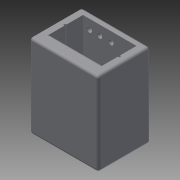
# Autodesk Inventor part: Part1
Saved by Autodesk Inventor 2014 SP1 (Build 180222100, 222)
## iProperties
Created: 2013-12-01
Part Number: Part1
Material: Generic
Document SubType Name: Modeling
Designer: Tim
Density: 1 g/cm^3
Appearance: Default
Author: Tim
Autodesk Inventor part; units mm, degrees
ref_plane "YZ Plane" through (0, 0, 0) normal (1, 0, 0) x (0, 1, 0)
ref_plane "XZ Plane" through (0, 0, 0) normal (0, 1, 0) x (-1, 0, 0)
ref_plane "XY Plane" through (0, 0, 0) normal (0, 0, 1) x (1, 0, 0)
sketch "Sketch1" plane through (0, 0, 0) normal (0, 1, 0) x (-1, 0, 0)
  line L0 (27.4909, -23.2831) -> (-26.5091, -23.2831)
  line L1 (-26.5091, -23.2831) -> (-26.5091, 42.2169)
  line L2 (-26.5091, 42.2169) -> (27.4909, 42.2169)
  line L3 (27.4909, 42.2169) -> (27.4909, -23.2831)
  point P0 (0, 0)
  dimension "d0" = 54
  dimension "d1" = 65.5
  constraints: 8 end point, 2 parallel, 1 horizontal, 1 perpendicular
  measures "d0" distance between parallel lines of L3 L1
  measures "d1" distance between parallel lines of L0 L2
extrude "Extrusion1" add sketch "Sketch1" along normal blind 41
sketch "Sketch2" plane through (-27.4909, 0, 42.2169) normal (0, 0, 1) x (1, 0, 0)
  line L0 (54, 0) -> (0, 0) projected
  line L1 (54, 0) -> (54, 41) projected
  line L2 (0, 41) -> (54, 41) projected
  line L3 (0, 0) -> (0, 41) projected
  line L4 (6, 36) -> (48, 36)
  line L5 (48, 36) -> (48, 5)
  line L6 (48, 5) -> (6, 5)
  line L7 (6, 5) -> (6, 36)
  line L8 (5, 23) -> (49, 23)
  line L9 (49, 23) -> (49, 21.5)
  line L10 (49, 21.5) -> (5, 21.5)
  line L11 (5, 21.5) -> (5, 23)
  point P0 (27.4909, 0)
  dimension "d4" = 42
  dimension "d5" = 31
  dimension "d6" = 5
  dimension "d7" = 6
  dimension "d8" = 6
  dimension "d9" = 1
  dimension "d10" = 1
  dimension "d11" = 13
  dimension "d12" = 1.5
  dimension "d13" = 5
  constraints: 16 end point, 4 parallel, 2 horizontal, 2 perpendicular
  measures "d4" distance between parallel lines of L5 L7
  measures "d5" distance between parallel lines of L6 L4
  measures "d6" distance between parallel lines of L4 L2
  measures "d7" distance between parallel lines of L1 L5
  measures "d8" distance between parallel lines of L3 L7
  measures "d9" distance between parallel lines of L7 L11
  measures "d10" distance between parallel lines of L9 L5
  measures "d11" distance between parallel lines of L4 L8
  measures "d12" distance between parallel lines of L8 L10
  measures "d13" distance between parallel lines of L0 L6
extrude "Extrusion2" cut sketch "Sketch2" against normal blind 60.5 contours L4 L5 L8 L7 | L8 L5 L10 L7 | L7 L10 L11 L8 | L8 L9 L10 L5 | L10 L5 L6 L7
sketch "Sketch3" plane through (0, 41, 0) normal (0, 1, 0) x (1, 0, 0)
  line L0 (26.5091, 23.2831) -> (-27.4909, 23.2831) projected
  line L1 (26.5091, -42.2169) -> (26.5091, 23.2831) projected
  line L2 (-7.9909, -6.7169) -> (19.5091, -6.7169)
  line L3 (19.5091, -6.7169) -> (19.5091, 16.2831)
  line L4 (19.5091, 16.2831) -> (-7.9909, 16.2831)
  line L5 (-7.9909, 16.2831) -> (-7.9909, -6.7169)
  point P0 (0, 0)
  dimension "d16" = 34.5
  dimension "d17" = 30
  dimension "d18" = 7
  dimension "d19" = 7
  constraints: 8 end point, 2 parallel, 1 horizontal, 1 perpendicular
  measures "d16" distance between parallel lines of L1 L5
  measures "d17" distance between parallel lines of L0 L2
  measures "d18" distance between parallel lines of L0 L4
  measures "d19" distance between parallel lines of L1 L3
extrude "Extrusion3" cut sketch "Sketch3" against normal blind 5
sketch "Sketch4" plane through (-21.4909, 5, 42.2169) normal (0, 1, 0) x (1, 0, 0)
  line L0 (0, 0) -> (0, 60.5) projected
  line L1 (0, 3) -> (42, 3)
  line L2 (42, 3) -> (42, 0)
  line L3 (42, 0) -> (0, 0)
  line L4 (0, 0) -> (0, 3)
  point P0 (21.4909, 42.2169)
  dimension "d22" = 3
  constraints: 8 end point, 2 parallel, 1 horizontal, 1 perpendicular, 1 point on line
  measures "d22" distance between parallel lines of L3 L1
extrude "Extrusion4" add sketch "Sketch4" along normal blind 5 separate body
sketch "Sketch5" plane through (0, 41, 0) normal (0, 1, 0) x (1, 0, 0)
  line L0 (26.5091, 23.2831) -> (-27.4909, 23.2831) projected
  line L1 (-27.4909, 23.2831) -> (-27.4909, -42.2169) projected
  circle A0 centre (-16.4909, -34.7169) radius 2
  circle A1 centre (-8.4909, -34.7169) radius 2
  circle A2 centre (0.5091, -34.7169) radius 2
  point P0 (0, 0)
  dimension "d25" = 11
  dimension "d26" = 19
  dimension "d27" = 28
  dimension "d30" = 58
  dimension "d31" = 58
  dimension "d32" = 58
  dimension "d33" = 4
  dimension "d34" = 4
  dimension "d35" = 4
  constraints: 3 centre point
  measures "d25" distance from line of L1 A0.centre
  measures "d26" distance from line of A1.centre L1
  measures "d27" distance from line of A2.centre L1
  measures "d30" distance from line of L0 A0.centre
  measures "d31" distance from line of L0 A1.centre
  measures "d32" distance from line of L0 A2.centre
  measures "d33" diameter of A1
  measures "d34" diameter of A2
  measures "d35" diameter of A0
extrude "Extrusion5" cut sketch "Sketch5" against normal blind 5 bodies 1
fillet "Fillet3" radius 2 1 edges at (26.5091, 20.5, -23.2831)
fillet "Fillet4" radius 2 1 edges at (-27.4909, 20.5, -23.2831)
fillet "Fillet5" radius 2 5 edges at (-0.4909, 41, -23.2831) (-26.9051, 41, -22.6973) (-27.4909, 41, 10.4669) (25.9233, 41, -22.6973) (26.5091, 41, 10.4669)
fillet "Fillet6" radius 2 5 edges at (-0.4909, 0, -23.2831) (25.9233, 0, -22.6973) (26.5091, 0, 10.4669) (-26.9051, 0, -22.6973) (-27.4909, 0, 10.4669)
fillet "Fillet7" radius 2 8 edges at (-27.4909, 20.5, 42.2169) (-26.9051, 40.4142, 42.2169) (-0.4909, 41, 42.2169) (25.9233, 40.4142, 42.2169) (26.5091, 20.5, 42.2169) (25.9233, 0.5858, 42.2169) (-0.4909, 0, 42.2169) (-26.9051, 0.5858, 42.2169)
fillet "Fillet9" radius 1 3 edges at (-10.4909, 41, 34.7169) (-1.4909, 41, 34.7169) (-18.4909, 41, 34.7169)
fillet "Fillet11" radius 2 1 edges at (-0.4909, 10, 42.2169)
sketch "Sketch6" plane through (24.5091, 39, -23.2831) normal (0, 0, -1) x (-1, 0, 0)
  line L0 (50, 0) -> (50, -37) projected
  line L1 (0, 0) -> (50, 0) projected
  line L2 (0, -37) -> (0, 0) projected
  line L3 (3, -10) -> (47, -10) construction
  line L4 (47, -10) -> (47, -27) construction
  line L5 (47, -27) -> (3, -27) construction
  line L6 (3, -27) -> (3, -10) construction
  line L7 (5.0416, -16.1395) -> (5.0416, -10.7613)
  line L8 (5.0416, -10.7613) -> (2.9951, -10.7613)
  line L9 (2.9951, -10.7613) -> (2.9951, -10.0395)
  line L10 (2.9951, -10.0395) -> (7.8988, -10.0395)
  line L11 (7.8988, -10.0395) -> (7.8988, -10.7613)
  line L12 (7.8988, -10.7613) -> (5.8523, -10.7613)
  line L13 (5.8523, -10.7613) -> (5.8523, -16.1395)
  line L14 (5.8523, -16.1395) -> (5.0416, -16.1395)
  line L15 (9.2434, -16.1395) -> (8.4722, -16.1395)
  line L16 (8.4722, -16.1395) -> (8.4722, -11.5621)
  line L17 (8.4722, -11.5621) -> (9.2434, -11.5621)
  line L18 (9.2434, -11.5621) -> (9.2434, -16.1395)
  line L19 (9.2977, -10.8008) -> (8.4228, -10.8008)
  line L20 (8.4228, -10.8008) -> (8.4228, -10)
  line L21 (8.4228, -10) -> (9.2977, -10)
  line L22 (9.2977, -10) -> (9.2977, -10.8008)
  spline S0 degree 2 poles (12.1945, -16.2434) (11.7199, -16.2434) (10.934, -15.9517) (10.6522, -15.6551) knots 0 0 0 1 2 2 2
  spline S1 degree 2 poles (10.6522, -15.6551) (10.3704, -15.3635) (10.059, -14.4638) (10.059, -13.8607) knots 0 0 0 1 2 2 2
  spline S2 degree 2 poles (10.059, -13.8607) (10.059, -13.2576) (10.3803, -12.3777) (10.6522, -12.0811) knots 0 0 0 1 2 2 2
  spline S3 degree 2 poles (10.6522, -12.0811) (10.9241, -11.7796) (11.7298, -11.4583) (12.1945, -11.4583) knots 0 0 0 1 2 2 2
  spline S4 degree 2 poles (12.1945, -11.4583) (12.5702, -11.4583) (13.2721, -11.6708) (13.544, -11.8092) knots 0 0 0 1 2 2 2
  line L23 (13.544, -11.8092) -> (13.544, -12.6743)
  line L24 (13.544, -12.6743) -> (13.4995, -12.6743)
  spline S5 degree 2 poles (13.4995, -12.6743) (13.4155, -12.6051) (13.1584, -12.4271) (12.9755, -12.3332) knots 0 0 0 1 2 2 2
  spline S6 degree 2 poles (12.9755, -12.3332) (12.8124, -12.2541) (12.3774, -12.1306) (12.1797, -12.1306) knots 0 0 0 1 2 2 2
  spline S7 degree 2 poles (12.1797, -12.1306) (11.5815, -12.1306) (10.8549, -13.0352) (10.8549, -13.8607) knots 0 0 0 1 2 2 2
  spline S8 degree 2 poles (10.8549, -13.8607) (10.8549, -14.6665) (11.5568, -15.5711) (12.1797, -15.5711) knots 0 0 0 1 2 2 2
  spline S9 degree 2 poles (12.1797, -15.5711) (12.5553, -15.5711) (13.2375, -15.2596) (13.4995, -15.0174) knots 0 0 0 1 2 2 2
  line L25 (13.4995, -15.0174) -> (13.544, -15.0174)
  line L26 (13.544, -15.0174) -> (13.544, -15.8825)
  spline S10 degree 2 poles (13.544, -15.8825) (13.4303, -15.9369) (13.0843, -16.0901) (12.9459, -16.1247) knots 0 0 0 1 2 2 2
  spline S11 degree 2 poles (12.9459, -16.1247) (12.7481, -16.184) (12.4367, -16.2434) (12.1945, -16.2434) knots 0 0 0 1 2 2 2
  line L27 (16.3666, -13.8409) -> (14.0581, -13.8409)
  line L28 (14.0581, -13.8409) -> (14.0581, -13.0994)
  line L29 (14.0581, -13.0994) -> (16.3666, -13.0994)
  line L30 (16.3666, -13.0994) -> (16.3666, -13.8409)
  line L31 (18.774, -16.1395) -> (18.774, -10.7613)
  line L32 (18.774, -10.7613) -> (16.7275, -10.7613)
  line L33 (16.7275, -10.7613) -> (16.7275, -10.0395)
  line L34 (16.7275, -10.0395) -> (21.6312, -10.0395)
  line L35 (21.6312, -10.0395) -> (21.6312, -10.7613)
  line L36 (21.6312, -10.7613) -> (19.5847, -10.7613)
  line L37 (19.5847, -10.7613) -> (19.5847, -16.1395)
  line L38 (19.5847, -16.1395) -> (18.774, -16.1395)
  spline S12 degree 2 poles (24.7405, -15.6551) (24.6466, -15.7243) (24.3302, -15.9715) (24.1819, -16.0456) knots 0 0 0 1 2 2 2
  spline S13 degree 2 poles (24.1819, -16.0456) (23.9793, -16.1544) (23.5986, -16.2681) (23.2526, -16.2681) knots 0 0 0 1 2 2 2
  spline S14 degree 2 poles (23.2526, -16.2681) (22.9708, -16.2681) (22.4617, -16.0555) (22.2689, -15.8627) knots 0 0 0 1 2 2 2
  spline S15 degree 2 poles (22.2689, -15.8627) (22.086, -15.6749) (21.8635, -15.1212) (21.8635, -14.8147) knots 0 0 0 1 2 2 2
  spline S16 degree 2 poles (21.8635, -14.8147) (21.8635, -14.3402) (22.2639, -13.6679) (22.6989, -13.4751) knots 0 0 0 1 2 2 2
  spline S17 degree 2 poles (22.6989, -13.4751) (23.0845, -13.2972) (24.1325, -13.1637) (24.7405, -13.1291) knots 0 0 0 1 2 2 2
  line L39 (24.7405, -13.1291) -> (24.7405, -12.9808)
  spline S18 degree 2 poles (24.7405, -12.9808) (24.7405, -12.7139) (24.5774, -12.3827) (24.4291, -12.2887) knots 0 0 0 1 2 2 2
  spline S19 degree 2 poles (24.4291, -12.2887) (24.2808, -12.1948) (23.8557, -12.1355) (23.6283, -12.1355) knots 0 0 0 1 2 2 2
  spline S20 degree 2 poles (23.6283, -12.1355) (23.3613, -12.1355) (22.6396, -12.2937) (22.2788, -12.4469) knots 0 0 0 1 2 2 2
  line L40 (22.2788, -12.4469) -> (22.2343, -12.4469)
  line L41 (22.2343, -12.4469) -> (22.2343, -11.6609)
  spline S21 degree 2 poles (22.2343, -11.6609) (22.4468, -11.6016) (23.2427, -11.4533) (23.6332, -11.4533) knots 0 0 0 1 2 2 2
  spline S22 degree 2 poles (23.6332, -11.4533) (24.1078, -11.4533) (24.7553, -11.6016) (25.0124, -11.7944) knots 0 0 0 1 2 2 2
  spline S23 degree 2 poles (25.0124, -11.7944) (25.2645, -11.9823) (25.5117, -12.5804) (25.5117, -13.0105) knots 0 0 0 1 2 2 2
  line L42 (25.5117, -13.0105) -> (25.5117, -16.1395)
  line L43 (25.5117, -16.1395) -> (24.7405, -16.1395)
  line L44 (24.7405, -16.1395) -> (24.7405, -15.6551)
  line L45 (24.7405, -15.0125) -> (24.7405, -13.7421)
  spline S24 degree 2 poles (24.7405, -13.7421) (24.4637, -13.7668) (23.6283, -13.8508) (23.3663, -13.9299) knots 0 0 0 1 2 2 2
  spline S25 degree 2 poles (23.3663, -13.9299) (23.0598, -14.0238) (22.6594, -14.4143) (22.6594, -14.7604) knots 0 0 0 1 2 2 2
  spline S26 degree 2 poles (22.6594, -14.7604) (22.6594, -15.1558) (23.1043, -15.5562) (23.5294, -15.5562) knots 0 0 0 1 2 2 2
  spline S27 degree 2 poles (23.5294, -15.5562) (23.8903, -15.5562) (24.4835, -15.2448) (24.7405, -15.0125) knots 0 0 0 1 2 2 2
  spline S28 degree 2 poles (28.4134, -16.2434) (27.9388, -16.2434) (27.1528, -15.9517) (26.8711, -15.6551) knots 0 0 0 1 2 2 2
  spline S29 degree 2 poles (26.8711, -15.6551) (26.5893, -15.3635) (26.2779, -14.4638) (26.2779, -13.8607) knots 0 0 0 1 2 2 2
  spline S30 degree 2 poles (26.2779, -13.8607) (26.2779, -13.2576) (26.5992, -12.3777) (26.8711, -12.0811) knots 0 0 0 1 2 2 2
  spline S31 degree 2 poles (26.8711, -12.0811) (27.143, -11.7796) (27.9487, -11.4583) (28.4134, -11.4583) knots 0 0 0 1 2 2 2
  spline S32 degree 2 poles (28.4134, -11.4583) (28.7891, -11.4583) (29.491, -11.6708) (29.7629, -11.8092) knots 0 0 0 1 2 2 2
  line L46 (29.7629, -11.8092) -> (29.7629, -12.6743)
  line L47 (29.7629, -12.6743) -> (29.7184, -12.6743)
  spline S33 degree 2 poles (29.7184, -12.6743) (29.6344, -12.6051) (29.3773, -12.4271) (29.1944, -12.3332) knots 0 0 0 1 2 2 2
  spline S34 degree 2 poles (29.1944, -12.3332) (29.0313, -12.2541) (28.5963, -12.1306) (28.3985, -12.1306) knots 0 0 0 1 2 2 2
  spline S35 degree 2 poles (28.3985, -12.1306) (27.8004, -12.1306) (27.0737, -13.0352) (27.0737, -13.8607) knots 0 0 0 1 2 2 2
  spline S36 degree 2 poles (27.0737, -13.8607) (27.0737, -14.6665) (27.7757, -15.5711) (28.3985, -15.5711) knots 0 0 0 1 2 2 2
  spline S37 degree 2 poles (28.3985, -15.5711) (28.7742, -15.5711) (29.4564, -15.2596) (29.7184, -15.0174) knots 0 0 0 1 2 2 2
  line L48 (29.7184, -15.0174) -> (29.7629, -15.0174)
  line L49 (29.7629, -15.0174) -> (29.7629, -15.8825)
  spline S38 degree 2 poles (29.7629, -15.8825) (29.6492, -15.9369) (29.3032, -16.0901) (29.1647, -16.1247) knots 0 0 0 1 2 2 2
  spline S39 degree 2 poles (29.1647, -16.1247) (28.967, -16.184) (28.6556, -16.2434) (28.4134, -16.2434) knots 0 0 0 1 2 2 2
  line L50 (32.5855, -13.8409) -> (30.277, -13.8409)
  line L51 (30.277, -13.8409) -> (30.277, -13.0994)
  line L52 (30.277, -13.0994) -> (32.5855, -13.0994)
  line L53 (32.5855, -13.0994) -> (32.5855, -13.8409)
  line L54 (34.9929, -16.1395) -> (34.9929, -10.7613)
  line L55 (34.9929, -10.7613) -> (32.9464, -10.7613)
  line L56 (32.9464, -10.7613) -> (32.9464, -10.0395)
  line L57 (32.9464, -10.0395) -> (37.8501, -10.0395)
  line L58 (37.8501, -10.0395) -> (37.8501, -10.7613)
  line L59 (37.8501, -10.7613) -> (35.8036, -10.7613)
  line L60 (35.8036, -10.7613) -> (35.8036, -16.1395)
  line L61 (35.8036, -16.1395) -> (34.9929, -16.1395)
  spline S40 degree 2 poles (42.1705, -13.8508) (42.1705, -15.0075) (41.0583, -16.2681) (40.1289, -16.2681) knots 0 0 0 1 2 2 2
  spline S41 degree 2 poles (40.1289, -16.2681) (39.1749, -16.2681) (38.0824, -14.968) (38.0824, -13.8508) knots 0 0 0 1 2 2 2
  spline S42 degree 2 poles (38.0824, -13.8508) (38.0824, -12.704) (39.2095, -11.4335) (40.1289, -11.4335) knots 0 0 0 1 2 2 2
  spline S43 degree 2 poles (40.1289, -11.4335) (41.0583, -11.4335) (42.1705, -12.699) (42.1705, -13.8508) knots 0 0 0 1 2 2 2
  spline S44 degree 2 poles (41.3746, -13.8508) (41.3746, -12.961) (40.7271, -12.0959) (40.1289, -12.0959) knots 0 0 0 1 2 2 2
  spline S45 degree 2 poles (40.1289, -12.0959) (39.5308, -12.0959) (38.8783, -12.961) (38.8783, -13.8508) knots 0 0 0 1 2 2 2
  spline S46 degree 2 poles (38.8783, -13.8508) (38.8783, -14.7159) (39.5308, -15.6057) (40.1289, -15.6057) knots 0 0 0 1 2 2 2
  spline S47 degree 2 poles (40.1289, -15.6057) (40.7221, -15.6057) (41.3746, -14.7307) (41.3746, -13.8508) knots 0 0 0 1 2 2 2
  spline S48 degree 2 poles (44.9486, -16.2434) (43.8512, -16.2434) (42.6451, -15.0125) (42.6451, -13.8755) knots 0 0 0 1 2 2 2
  spline S49 degree 2 poles (42.6451, -13.8755) (42.6451, -12.7583) (43.8166, -11.4335) (44.7608, -11.4335) knots 0 0 0 1 2 2 2
  spline S50 degree 2 poles (44.7608, -11.4335) (45.1859, -11.4335) (45.8434, -11.6807) (46.0856, -11.9427) knots 0 0 0 1 2 2 2
  spline S51 degree 2 poles (46.0856, -11.9427) (46.3327, -12.2047) (46.5947, -12.961) (46.5947, -13.5097) knots 0 0 0 1 2 2 2
  line L62 (46.5947, -13.5097) -> (46.5947, -13.9299)
  line L63 (46.5947, -13.9299) -> (43.4261, -13.9299)
  spline S52 degree 2 poles (43.4261, -13.9299) (43.4261, -14.7258) (44.2269, -15.5711) (44.9387, -15.5711) knots 0 0 0 1 2 2 2
  spline S53 degree 2 poles (44.9387, -15.5711) (45.1908, -15.5711) (45.6802, -15.4574) (45.878, -15.3684) knots 0 0 0 1 2 2 2
  spline S54 degree 2 poles (45.878, -15.3684) (46.0856, -15.2695) (46.3723, -15.0965) (46.4662, -15.0174) knots 0 0 0 1 2 2 2
  line L64 (46.4662, -15.0174) -> (46.5107, -15.0174)
  line L65 (46.5107, -15.0174) -> (46.5107, -15.8578)
  spline S55 degree 2 poles (46.5107, -15.8578) (46.3772, -15.9122) (45.9719, -16.0703) (45.8137, -16.1148) knots 0 0 0 1 2 2 2
  spline S56 degree 2 poles (45.8137, -16.1148) (45.5912, -16.1791) (45.2254, -16.2434) (44.9486, -16.2434) knots 0 0 0 1 2 2 2
  spline S57 degree 2 poles (45.8434, -13.3417) (45.8335, -13.0302) (45.7049, -12.5754) (45.5814, -12.4222) knots 0 0 0 1 2 2 2
  spline S58 degree 2 poles (45.5814, -12.4222) (45.4479, -12.2492) (45.0277, -12.0663) (44.7163, -12.0663) knots 0 0 0 1 2 2 2
  spline S59 degree 2 poles (44.7163, -12.0663) (44.4098, -12.0663) (43.9797, -12.2492) (43.8018, -12.4271) knots 0 0 0 1 2 2 2
  spline S60 degree 2 poles (43.8018, -12.4271) (43.6288, -12.61) (43.4508, -13.05) (43.4261, -13.3417) knots 0 0 0 1 2 2 2
  line L66 (43.4261, -13.3417) -> (45.8434, -13.3417)
  line L67 (5.0416, -26.183) -> (5.0416, -20.8048)
  line L68 (5.0416, -20.8048) -> (2.9951, -20.8048)
  line L69 (2.9951, -20.8048) -> (2.9951, -20.083)
  line L70 (2.9951, -20.083) -> (7.8988, -20.083)
  line L71 (7.8988, -20.083) -> (7.8988, -20.8048)
  line L72 (7.8988, -20.8048) -> (5.8523, -20.8048)
  line L73 (5.8523, -20.8048) -> (5.8523, -26.183)
  line L74 (5.8523, -26.183) -> (5.0416, -26.183)
  line L75 (9.6536, -26.183) -> (8.6749, -26.183)
  line L76 (8.6749, -26.183) -> (8.6749, -25.0164)
  line L77 (8.6749, -25.0164) -> (9.6536, -25.0164)
  line L78 (9.6536, -25.0164) -> (9.6536, -26.183)
  line L79 (15.4867, -26.183) -> (14.676, -26.183)
  line L80 (14.676, -26.183) -> (14.676, -23.1973)
  line L81 (14.676, -23.1973) -> (11.8682, -23.1973)
  line L82 (11.8682, -23.1973) -> (11.8682, -26.183)
  line L83 (11.8682, -26.183) -> (11.0575, -26.183)
  line L84 (11.0575, -26.183) -> (11.0575, -20.083)
  line L85 (11.0575, -20.083) -> (11.8682, -20.083)
  line L86 (11.8682, -20.083) -> (11.8682, -22.4756)
  line L87 (11.8682, -22.4756) -> (14.676, -22.4756)
  line L88 (14.676, -22.4756) -> (14.676, -20.083)
  line L89 (14.676, -20.083) -> (15.4867, -20.083)
  line L90 (15.4867, -20.083) -> (15.4867, -26.183)
  line L91 (17.8595, -26.183) -> (16.8807, -26.183)
  line L92 (16.8807, -26.183) -> (16.8807, -25.0164)
  line L93 (16.8807, -25.0164) -> (17.8595, -25.0164)
  line L94 (17.8595, -25.0164) -> (17.8595, -26.183)
  point P0 (24.5091, -39)
  dimension "d49" = 3
  dimension "d50" = 3
  dimension "d51" = 10
  dimension "d52" = 17
  constraints: 2 other
  measures "d49" distance between parallel lines of L2 L6
  measures "d50" distance between parallel lines of L0 L4
  measures "d51" distance between parallel lines of L1 L3
  measures "d52" distance between parallel lines of L3 L5
extrude "Extrusion6" cut sketch "Sketch6" against normal blind 1 bodies 1
combine bodies "Combine1" operation type add bodies to combine 2 1
fillet "Fillet12" radius 5 1 edges at (-0.4909, 5, 39.2169)
chamfer "Chamfer1" distance 4 angle 45 4 edges at (19.5091, 38.5, -16.2831) (-7.9909, 38.5, -16.2831) (-7.9909, 38.5, 6.7169) (19.5091, 38.5, 6.7169)
fillet "Fillet16" radius 2 8 edges at (5.7591, 41, -16.2831) (-5.9909, 41, -14.2831) (-7.9909, 41, -4.7831) (-5.9909, 41, 4.7169) (5.7591, 41, 6.7169) (17.5091, 41, 4.7169) (19.5091, 41, -4.7831) (17.5091, 41, -14.2831)
equation "\"d31\" = d30"
equation "\"d32\" = d30"
equation "\"d34\" = d33"
equation "\"d35\" = d33"
body "Solid2"
